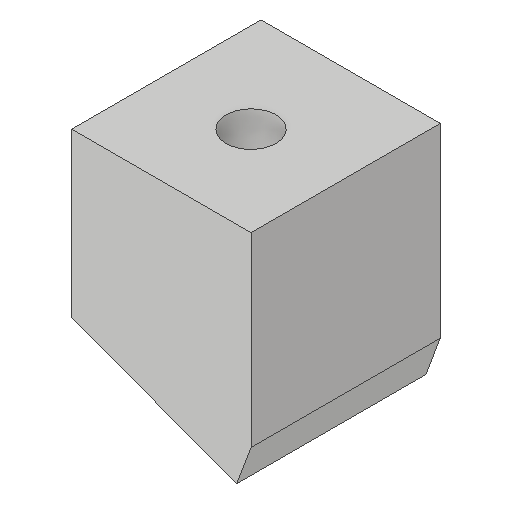
# Autodesk Inventor part: 3DP_PLA_Measurement_Rail_Rammer
Saved by Autodesk Inventor 2025 (Build 290162010, 162A)
## iProperties
Created: 2018-06-15
Part Number: 3DP_PLA_Measurement_Rail_Rammer
Material: Generic
Document SubType Name: Modeling
Designer: Andrzej
Density: 1 g/cm^3
Appearance: Default
Author: Andrzej
Autodesk Inventor part; units mm, degrees
ref_plane "YZ Plane" through (0, 0, 0) normal (1, 0, 0) x (0, 1, 0)
ref_plane "XZ Plane" through (0, 0, 0) normal (0, 1, 0) x (-1, 0, 0)
ref_plane "XY Plane" through (0, 0, 0) normal (0, 0, 1) x (1, 0, 0)
sketch "Sketch2" plane through (0, 0, 0) normal (0, 0, 1) x (1, 0, 0)
  line L0 (-5.0655, 3.6572) -> (12.9345, 3.6572)
  line L1 (12.9345, 3.6572) -> (12.9345, -8.3428)
  line L2 (12.9345, -8.3428) -> (-5.0655, -8.3428)
  line L3 (-5.0655, -8.3428) -> (-5.0655, 3.6572)
  line L4 (8.9345, 3.6572) -> (7.7095, 0.3786)
  line L5 (7.7095, 0.3786) -> (-1.0655, 3.6572)
  line L6 (-1.0655, 3.6572) -> (-1.0655, 11.6572)
  line L7 (-1.0655, 11.6572) -> (8.9345, 11.6572)
  line L8 (8.9345, 11.6572) -> (8.9345, 3.6572)
  point P0 (0, 0)
  dimension "d0" = 18
  dimension "d1" = 12
  dimension "d2" = 3.5
  dimension "d3" = 4
  dimension "d4" = 4
  dimension "d5" = 110.487
  dimension "d6" = 8
  constraints: 18 end point, 4 perpendicular, 2 parallel, 2 point on line, 1 horizontal, 1 vertical
  measures "d0" distance of L1.end L2.end
  measures "d1" distance of L0.end L1.end
  measures "d2" distance of L4.start L4.end
  measures "d3" distance from line of L3 L5.end
  measures "d4" distance of L0.end L4.start
  measures "d5" angle of L0 L4
  measures "d6" distance of L5.end L6.end
extrude "Extrusion1" add sketch "Sketch2" along normal blind 9.5 contours L6 L7 L8 L0 | L0 L4 L5
sketch "Sketch3" plane through (0, 0, 9.5) normal (0, 0, 1) x (1, 0, 0)
  line L0 (-1.0655, 3.6572) -> (7.7095, 0.3786) projected
  line L1 (7.7095, 0.3786) -> (8.9345, 3.6572) projected
  line L2 (8.9345, 3.6572) -> (8.9345, 11.6572) projected
  line L3 (8.9345, 11.6572) -> (-1.0655, 11.6572) projected
  line L4 (-1.0655, 11.6572) -> (-1.0655, 3.6572) projected
  line L5 (-0.5655, 15.4431) -> (8.4345, 15.4431)
  line L6 (8.4345, 15.4431) -> (8.4345, -6.1671)
  line L7 (8.4345, -6.1671) -> (-0.5655, -6.1671)
  line L8 (-0.5655, -6.1671) -> (-0.5655, 15.4431)
  point P0 (0, 0)
  dimension "d9" = 0.5
  dimension "d10" = 0.5
  constraints: 8 end point, 2 parallel, 1 horizontal, 1 perpendicular
  measures "d9" distance between parallel lines of L4 L8
  measures "d10" distance between parallel lines of L2 L6
extrude "Extrusion2" cut sketch "Sketch3" against normal blind 10 contours L8 L3 L6 L1 L0 | L0 L1 L6 L7 L8 | L8 L5 L6 L3 keep common part
sketch "Sketch4" plane through (-0.5655, 11.6572, 9.5) normal (0, 1, 0) x (1, 0, 0)
  line L0 (0, 0) -> (0, 9.5) projected
  line L1 (9, 0) -> (0, 0) projected
  line L2 (9, 9.5) -> (9, 0) projected
  line L3 (9, 9.5) -> (0, 9.5) projected
  point P0 (0.5655, 9.5)
  point P1 (4.5, 4.5)
  dimension "d13" = 4.5
  dimension "d14" = 4.5
  dimension "d15" = 9
  dimension "d16" = 9.5
  measures "d13" distance from line of L1 point (4.5, 4.5)
  measures "d14" distance from line of L2 point (4.5, 4.5)
  measures "d15" distance between parallel lines of L2 L0
  measures "d16" distance of L2.start L1.start
hole "Hole1" at (3.9345, 11.6572, 5) direction (0, -1, 0) diameter 2.5 depth 7 tip angle 118
equation "\"d14\" = 0.5 * d15"
body "Solid1"
